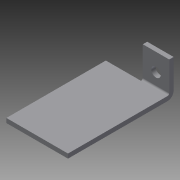
# Autodesk Inventor part: pawl mount
Saved by Autodesk Inventor 2013 (Build 170138000, 138)
## iProperties
Created: 2013-02-05
Part Number: pawl mount
Material: Generic
Document SubType Name: Sheet Metal
Designer: Arpan
Density: 1 g/cm^3
Sheet Metal Rule: Default
Author: Arpan
Autodesk Inventor part; units mm, degrees
ref_plane "YZ Plane" through (0, 0, 0) normal (1, 0, 0) x (0, 1, 0)
ref_plane "XZ Plane" through (0, 0, 0) normal (0, 1, 0) x (-1, 0, 0)
ref_plane "XY Plane" through (0, 0, 0) normal (0, 0, 1) x (1, 0, 0)
sketch "Sketch1" plane through (0, 0, 0) normal (0, 0, 1) x (1, 0, 0)
  circle A0 centre (9.525, -12.7) radius 3.3782
  line L0 (19.05, 0) -> (0, 0)
  line L1 (0, 0) -> (0, -25.4)
  line L2 (19.05, -25.4) -> (0, -25.4)
  line L3 (19.05, 0) -> (19.05, -25.4)
extrude "Plate1" add sketch "Sketch1" along normal blind 3.175
sketch "Sketch2" plane through (19.05, -22.225, 0) normal (0, -1, 0) x (1, 0, 0)
  line L0 (-19.05, 0) -> (0, 0)
  line L1 (0, 0) -> (0, 25.4)
  line L2 (0, 25.4) -> (-19.05, 25.4)
  line L3 (-19.05, 25.4) -> (-19.05, 0)
  constraints: 6 end point, 1 horizontal, 1 perpendicular, 1 vertical
edge flange "Flange1" height 25.4 angle 90 thickness 3.175 bend radius 1.27 thickness toward (0, -1, 0) relief tear relief width 3.175 relief depth 1.5875 edges at (9.525, -25.4, 3.175) wall of the first edge with corners at (0, -22.225, 0) (19.05, -22.225, 0) (19.05, -22.225, 25.4) (0, -22.225, 25.4)
bend "Bend1"
corner "Corner1"
sketch "Sketch3" plane through (0, -25.4, 25.4) normal (0, 0, 1) x (1, 0, 0)
  line L0 (0, 0) -> (19.05, 0) projected
  line L1 (19.05, 3.175) -> (19.05, 0) projected
  line L2 (0, 3.175) -> (19.05, 3.175) projected
  line L3 (0, 3.175) -> (0, 0) projected
  point P0 (0, 25.4)
extrude "Extrusion1" add sketch "Sketch3" along normal blind 50.8
sketch "Sketch5" plane through (0, -25.4, 4.445) normal (-1, 0, 0) x (0, 0, 1)
  line L0 (0, 3.175) -> (0, 0) projected
  line L1 (0, 0) -> (71.755, 0) projected
  line L2 (71.755, 3.175) -> (71.755, 0) projected
  line L3 (71.755, 3.175) -> (0, 3.175) projected
  point P0 (-4.445, 25.4)
extrude "Extrusion3" add sketch "Sketch5" along normal blind 25.4
equation "\"d1\" = BendReliefWidth"
equation "\"d2\" = BendReliefDepth"
equation "\"d3\" = MinimumRemnant"
equation "\"d4\" = BendRadius"
equation "\"d8\" = CornerReliefSize"
equation "\"d9\" = GapSize"
equation "\"d10\" = JacobiRadiusSize"
equation "\"BendRadius\" = Thickness"
equation "\"BendReliefWidth\" = Thickness"
equation "\"BendReliefDepth\" = 0.5 * Thickness"
equation "\"CornerReliefSize\" = 4 * Thickness"
equation "\"MinimumRemnant\" = 2 * Thickness"
equation "\"TransitionRadius\" = BendRadius"
equation "\"JacobiRadiusSize\" = Thickness"
equation "\"GapSize\" = Thickness"
equation "\"d0\" = BendRadius"
equation "\"Thickness\" = 3.175"
body "Solid1"
